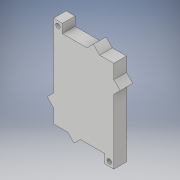
# Autodesk Inventor part: cage
Saved by Autodesk Inventor 2019 (Build 230136000, 136)
## iProperties
Created: 2021-05-02
Part Number: cage
Material: Generisch
Document SubType Name: Modeling
Designer: Michael Hohenstein
Density: 1 g/cm^3
Appearance: Vorgabe
Author: Michael Hohenstein
Autodesk Inventor part; units mm, degrees
ref_plane "YZ Plane" through (0, 0, 0) normal (1, 0, 0) x (0, 1, 0)
ref_plane "XZ Plane" through (0, 0, 0) normal (0, 1, 0) x (-1, 0, 0)
ref_plane "XY Plane" through (0, 0, 0) normal (0, 0, 1) x (1, 0, 0)
sketch "Skizze1" plane through (0, 0, 0) normal (0, 0, 1) x (1, 0, 0)
  line L0 (-17.75, -25.25) -> (17.75, -25.25)
  line L1 (17.75, -25.25) -> (17.75, 25.25)
  line L2 (17.75, 25.25) -> (-17.75, 25.25)
  line L3 (-17.75, 25.25) -> (-17.75, -25.25)
  line L4 (20.25, 27.75) -> (20.25, -27.75)
  line L5 (20.25, -27.75) -> (-20.25, -27.75)
  line L6 (-20.25, -27.75) -> (-20.25, 27.75)
  line L7 (-20.25, 27.75) -> (20.25, 27.75)
  point P0 (0, 0)
  point P1 (0, 25.25)
  point P2 (17.75, 0)
  dimension "d0" = 50.5
  dimension "d1" = 35.5
  dimension "d2" = 2.5
  constraints: 16 end point, 4 parallel, 2 midpoint, 2 perpendicular, 1 horizontal, 1 horizontal alignment, 1 vertical alignment, 3 other
  measures "d0" distance of L0.end L1.end
  measures "d1" distance of L1.end L2.end
  measures "d2" distance between parallel lines of L1 L4
extrude "Extrusion1" [suppressed]
extrude "Extrusion2" add sketch "Skizze1" along normal blind 6
sketch "Skizze2" plane through (0, 0, -2.5) normal (0, 0, -1) x (-1, 0, 0)
  circle A0 centre (0, 0) radius 1.5
  dimension "d7" = 3
  constraints: 1 centre point, 1 coincident
  measures "d7" diameter of A0
extrude "Extrusion3" [suppressed]
sketch "Skizze3" plane through (0, 0, 6) normal (0, 0, 1) x (1, 0, 0)
  line L0 (2.2647, 27.75) -> (10.75, 27.75)
  line L1 (10.75, 27.75) -> (6.5074, 31.9926)
  line L2 (6.5074, 31.9926) -> (2.2647, 27.75)
  line L3 (20.25, 18.25) -> (20.25, 9.7647)
  line L4 (20.25, 9.7647) -> (24.4926, 14.0074)
  line L5 (24.4926, 14.0074) -> (20.25, 18.25)
  line L6 (20.25, 27.75) -> (-20.25, 27.75) projected
  line L7 (20.25, -27.75) -> (20.25, 27.75) projected
  line L8 (4.386, 29.8713) -> (22.3713, 11.886) construction
  line L9 (-20.25, -9.7647) -> (-20.25, -18.25)
  line L10 (-20.25, -18.25) -> (-24.4926, -14.0074)
  line L11 (-24.4926, -14.0074) -> (-20.25, -9.7647)
  line L12 (-10.75, -27.75) -> (-2.2647, -27.75)
  line L13 (-2.2647, -27.75) -> (-6.5074, -31.9926)
  line L14 (-6.5074, -31.9926) -> (-10.75, -27.75)
  line L15 (-20.25, 27.75) -> (-20.25, -27.75) projected
  line L16 (-20.25, -27.75) -> (20.25, -27.75) projected
  line L17 (-22.3713, -11.886) -> (-4.386, -29.8713) construction
  line L18 (17.75, 25.25) -> (17.75, -25.25) projected
  line L19 (-17.75, -25.25) -> (-17.75, 25.25) projected
  line L20 (-17.75, 25.25) -> (17.75, 25.25) projected
  line L21 (17.75, -25.25) -> (-17.75, -25.25) projected
  point P0 (0, 0)
  dimension "d11" = 6
  dimension "d26" = 7
  dimension "d27" = 7
  constraints: 28 end point, 10 equal length, 4 midpoint, 4 point on line, 2 horizontal, 2 perpendicular, 2 vertical, 1 parallel
  measures "d11" distance of L0.end L1.end
  measures "d26" distance from line of L3.start L20
  measures "d27" distance from line of L9.end L21
extrude "Extrusion4" add sketch "Skizze3" against normal blind 6 contours L2 L1 L0 | L9 L10 L11 | L5 L4 L3 | L12 L13 L14
sketch "Skizze4" plane through (6.5074, 31.9926, 0) normal (-0.7071, 0.7071, 0) x (-0.7071, -0.7071, 0)
  circle A0 centre (3, 3) radius 1.65
  line L0 (6, 0) -> (6, 6) construction
  line L1 (0, 6) -> (0, 0) construction
  line L2 (6, 0) -> (0, 0) construction
  line L3 (0, 0) -> (0, 6) construction
  line L4 (0, 6) -> (6, 6) construction
  line L5 (6, 6) -> (6, 0) construction
  point P0 (27.2236, 0)
  point P1 (0, 3)
  point P2 (3, 0)
  dimension "d28" = 3.3
  constraints: 8 end point, 2 midpoint, 2 parallel, 1 centre point, 1 horizontal, 1 horizontal alignment, 1 perpendicular, 1 vertical alignment
  measures "d28" diameter of A0
extrude "Extrusion5" cut sketch "Skizze4" against normal up to surface (25.435 mm away)
sketch "Skizze7" plane through (-20.25, -9.7647, 0) normal (-0.7071, 0.7071, 0) x (-0.7071, -0.7071, 0)
  line L0 (0, 0) -> (0, 6) construction
  line L1 (6, 6) -> (6, 0) construction
  line L2 (0, 0) -> (6, 0) construction
  line L3 (6, 0) -> (6, 6) construction
  line L4 (6, 6) -> (0, 6) construction
  line L5 (0, 6) -> (0, 0) construction
  circle A0 centre (3, 3) radius 1.65
  point P0 (-21.2236, 0)
  point P1 (0, 3)
  point P2 (3, 6)
  dimension "d29" = 3.3
  constraints: 8 end point, 2 midpoint, 2 parallel, 1 centre point, 1 horizontal, 1 horizontal alignment, 1 perpendicular, 1 vertical alignment
  measures "d29" diameter of A0
extrude "Extrusion8" cut sketch "Skizze7" against normal up to surface (25.435 mm away)
sketch "Skizze8" plane through (0, 0, 6) normal (0, 0, 1) x (1, 0, 0)
  line L0 (-20.25, 27.75) -> (2.2647, 27.75) projected
  line L1 (-20.25, 27.75) -> (-20.25, -9.7647)
  line L2 (-20.25, -9.7647) -> (-24.4926, -14.0074) projected
  line L3 (-20.25, -9.7647) -> (-24.4926, -14.0074)
  line L4 (-24.4926, -14.0074) -> (-20.25, -18.25)
  line L5 (-10.75, -27.75) -> (-20.25, -27.75) projected
  line L6 (-20.25, -18.25) -> (-20.25, -27.75)
  line L7 (-20.25, -27.75) -> (-10.75, -27.75)
  line L8 (-10.75, -27.75) -> (-6.5074, -31.9926) projected
  line L9 (-10.75, -27.75) -> (-6.5074, -31.9926)
  line L10 (-2.2647, -27.75) -> (-6.5074, -31.9926) projected
  line L11 (-6.5074, -31.9926) -> (-2.2647, -27.75)
  line L12 (-2.2647, -27.75) -> (20.25, -27.75) projected
  line L13 (-2.2647, -27.75) -> (20.25, -27.75)
  line L14 (20.25, 9.7647) -> (20.25, -27.75) projected
  line L15 (20.25, -27.75) -> (20.25, 9.7647)
  line L16 (24.4926, 14.0074) -> (20.25, 9.7647) projected
  line L17 (20.25, 9.7647) -> (24.4926, 14.0074)
  line L18 (20.25, 27.75) -> (20.25, 18.25) projected
  line L19 (24.4926, 14.0074) -> (20.25, 18.25)
  line L20 (20.25, 18.25) -> (20.25, 27.75)
  line L21 (10.75, 27.75) -> (20.25, 27.75) projected
  line L22 (20.25, 27.75) -> (10.75, 27.75)
  line L23 (2.2647, 27.75) -> (6.5074, 31.9926) projected
  line L24 (10.75, 27.75) -> (6.5074, 31.9926)
  line L25 (6.5074, 31.9926) -> (2.2647, 27.75)
  line L26 (2.2647, 27.75) -> (-20.25, 27.75)
  point P0 (0, 0)
  constraints: 32 end point, 7 perpendicular, 6 collinear, 2 parallel, 1 vertical
extrude "Extrusion9" add sketch "Skizze8" along normal blind 2.5
sketch "Skizze11" plane through (0, 0, 8.5) normal (0, 0, 1) x (1, 0, 0)
  line L0 (-10.75, -27.75) -> (-20.25, -27.75) construction
  line L1 (20.25, 27.75) -> (20.25, 18.25) construction
  line L2 (-20.25, 27.75) -> (2.2647, 27.75) projected
  line L3 (-20.25, 27.75) -> (-14.25, 27.75)
  line L4 (-14.25, 27.75) -> (-14.25, 33.75)
  line L5 (-14.25, 33.75) -> (-20.25, 33.75)
  line L6 (-20.25, 33.75) -> (-20.25, 27.75)
  circle A0 centre (-17.25, 30.75) radius 1.5
  line L7 (20.25, -27.75) -> (-2.2647, -27.75) projected
  line L8 (20.25, -27.75) -> (14.25, -27.75)
  line L9 (14.25, -27.75) -> (14.25, -33.75)
  line L10 (14.25, -33.75) -> (20.25, -33.75)
  line L11 (20.25, -33.75) -> (20.25, -27.75)
  circle A1 centre (17.25, -30.75) radius 1.5
  point P0 (0, 0)
  point P1 (-20.25, 30.75)
  point P2 (-17.25, 33.75)
  point P3 (17.25, -27.75)
  point P4 (20.25, -30.75)
  dimension "d42" = 6
  dimension "d43" = 3
  constraints: 16 end point, 4 midpoint, 4 parallel, 3 equal length, 2 centre point, 2 horizontal, 2 horizontal alignment, 2 perpendicular, 2 vertical alignment, 1 equal radius
  measures "d42" distance of L4.end L5.end
  measures "d43" diameter of A0
extrude "Extrusion12" add sketch "Skizze11" against normal up to surface (8.5 mm away)
equation "\"d27\" = d26"
